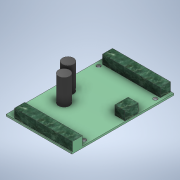
# Autodesk Inventor part: Switch Mode PS PCB
Saved by Autodesk Inventor 2021 (Build 250183000, 183)
## iProperties
Created: 2020-07-15
Part Number: Switch Mode PS PCB
Material: Generic
Document SubType Name: Modeling
Designer: jgray
Density: 1 g/cm^3
Appearance: Default
Author: jgray
Autodesk Inventor part; units mm, degrees
ref_plane "YZ Plane" through (0, 0, 0) normal (1, 0, 0) x (0, 1, 0)
ref_plane "XZ Plane" through (0, 0, 0) normal (0, 1, 0) x (-1, 0, 0)
ref_plane "XY Plane" through (0, 0, 0) normal (0, 0, 1) x (1, 0, 0)
sketch "Sketch1" plane through (0, 0, 0) normal (0, 1, 0) x (-1, 0, 0)
  line L0 (0, 0) -> (59, 0)
  line L1 (59, 0) -> (59, -91.5)
  line L2 (59, -91.5) -> (0, -91.5)
  line L3 (0, -91.5) -> (0, 0)
  line L4 (4, -15) -> (55, -15) construction
  line L5 (55, -15) -> (55, -79) construction
  line L6 (55, -79) -> (4, -79) construction
  line L7 (4, -79) -> (4, -15) construction
  dimension "d0" = 59
  dimension "d1" = 91.5
  dimension "d2" = 51
  dimension "d3" = 64
  dimension "d4" = 12.5
  dimension "d5" = 4
  constraints: 16 end point, 4 coincident, 4 parallel, 2 horizontal, 2 perpendicular
  measures "d0" distance of L1.end L2.end
  measures "d1" distance of L0.end L1.end
  measures "d2" distance of L5.end L6.end
  measures "d3" distance of L4.end L5.end
  measures "d4" distance between parallel lines of L2 L6
  measures "d5" distance between parallel lines of L3 L7
extrude "Extrusion1" add sketch "Sketch1" along normal blind 1.6
hole "Hole1" at (-55, 0, -15) at (-55, 0, -79) at (-4, 0, -79) at (-4, 0, -15) direction (0, 1, 0) diameter 3.5 end through all
sketch "Sketch2" plane through (0, 1.6, 0) normal (0, 1, 0) x (1, 0, 0)
  circle A0 centre (-49.5, 46) radius 5
  circle A1 centre (-42, 35) radius 5
  line L0 (-59, 0) -> (0, 0) projected
  line L1 (-59, 91.5) -> (-59, 0) projected
  line L2 (-52, 0.5) -> (0, 0.5)
  line L3 (0, 0.5) -> (0, 9.5)
  line L4 (0, 9.5) -> (-52, 9.5)
  line L5 (-52, 9.5) -> (-52, 0.5)
  line L6 (-54.5, 82) -> (-2.5, 82)
  line L7 (-2.5, 82) -> (-2.5, 91)
  line L8 (-2.5, 91) -> (-54.5, 91)
  line L9 (-54.5, 91) -> (-54.5, 82)
  line L10 (-9.5, 48) -> (-0.5, 48)
  line L11 (-0.5, 48) -> (-0.5, 60)
  line L12 (-0.5, 60) -> (-9.5, 60)
  line L13 (-9.5, 60) -> (-9.5, 48)
  line L14 (0, 0) -> (0, 91.5) projected
  dimension "d15" = 10
  dimension "d16" = 10
  dimension "d18" = 46
  dimension "d19" = 9.5
  dimension "d20" = 35
  dimension "d21" = 17
  dimension "d22" = 52
  dimension "d23" = 9
  dimension "d24" = 7
  dimension "d25" = 9.5
  dimension "d26" = 52
  dimension "d27" = 9
  dimension "d28" = 9.5
  dimension "d29" = 4.5
  dimension "d30" = 9
  dimension "d31" = 12
  dimension "d32" = 9.5
  dimension "d33" = 48
  constraints: 24 end point, 6 parallel, 3 horizontal, 3 perpendicular, 2 centre point
  measures "d15" diameter of A0
  measures "d16" diameter of A1
  measures "d18" distance from line of L0 A0.centre
  measures "d19" distance from line of L1 A0.centre
  measures "d20" distance from line of L0 A1.centre
  measures "d21" distance from line of L1 A1.centre
  measures "d22" distance of L4.end L3.end
  measures "d23" distance of L3.end L2.end
  measures "d24" distance between parallel lines of L1 L5
  measures "d25" distance between parallel lines of L0 L4
  measures "d26" distance of L8.end L7.end
  measures "d27" distance of L7.end L6.end
  measures "d28" distance from line of L1.start L6
  measures "d29" distance between parallel lines of L1 L9
  measures "d30" distance of L12.end L11.end
  measures "d31" distance of L11.end L10.end
  measures "d32" distance between parallel lines of L14 L13
  measures "d33" distance between parallel lines of L0 L10
extrude "Extrusion2" add sketch "Sketch2" along normal blind 23 contours A0 | A1
extrude "Extrusion3" add sketch "Sketch2" along normal blind 8 contours L5 L4 L3 L2 | L9 L8 L7 L6 | L13 L12 L11 L10
body "Solid1"
